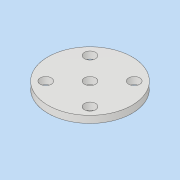
# Autodesk Inventor part: ServoHornDisc
Saved by Autodesk Inventor 2017.3 (Build 213256000, 256)
## iProperties
Created: 2016-11-02
Part Number: ServoHornDisc
Material: ABS Plastic
Document SubType Name: Modeling
Designer: techn
Density: 1.06 g/cm^3
Appearance: Smooth - White
Author: techn
Autodesk Inventor part; units mm, degrees
ref_plane "YZ Plane" through (0, 0, 0) normal (1, 0, 0) x (0, 1, 0)
ref_plane "XZ Plane" through (0, 0, 0) normal (0, 1, 0) x (-1, 0, 0)
ref_plane "XY Plane" through (0, 0, 0) normal (0, 0, 1) x (1, 0, 0)
sketch "Sketch1" plane through (0, 0, 0) normal (0, 1, 0) x (-1, 0, 0)
  circle A0 centre (0, 0) radius 2.8702
  dimension "d0" = 5.7404
  constraints: 1 centre point, 1 coincident
  measures "d0" diameter of A0
extrude "Extrusion1" add sketch "Sketch1" along normal blind 3.4036
sketch "Sketch6" plane through (0, 3.4036, 0) normal (0, 1, 0) x (1, 0, 0)
  circle A0 centre (0, 0) radius 11.938
  dimension "d22" = 23.876
  constraints: 1 centre point, 1 coincident
  measures "d22" diameter of A0
extrude "Extrusion8" add sketch "Sketch6" along normal mid plane 1.9939
sketch "Sketch7" plane through (0, 2.4067, 0) normal (0, -1, 0) x (1, 0, 0)
  circle A0 centre (0, 0) radius 4.445
  circle A1 centre (0, 0) radius 2.8702 projected
  circle A2 centre (0, 0) radius 1.5875
  dimension "d25" = 8.89
  dimension "d26" = 3.175
  constraints: 2 centre point, 2 coincident
  measures "d25" diameter of A0
  measures "d26" diameter of A2
extrude "Extrusion9" add sketch "Sketch7" along normal up to surface (2.4067 mm away) contours A0
extrude "Extrusion10" cut sketch "Sketch7" along normal through all contours A1 | A2
extrude "Extrusion11" cut sketch "Sketch7" against normal blind 1.9939 contours A2
sketch "Sketch8" plane through (0, 4.4006, 0) normal (0, 1, 0) x (1, 0, 0)
  line L0 (0, 0) -> (-6.2862, 6.2862)
  line L1 (0, 0) -> (8.89, 0) construction
  circle A0 centre (-6.2862, 6.2862) radius 1.5875
  circle A1 centre (-6.2862, -6.2862) radius 1.5875
  circle A2 centre (6.2862, -6.2862) radius 1.5875
  circle A3 centre (6.2862, 6.2862) radius 1.5875
  dimension "d33" = 8.89
  dimension "d34" = 135
  dimension "d35" = 3.175
  dimension "d38" = 360
  constraints: 4 centre point, 4 end point, 1 coincident, 1 equal length, 1 horizontal, 9 other
  measures "d33" distance of L0.start L0.end
  measures "d34" angle of L1 L0
  measures "d35" diameter of A0
extrude "Extrusion12" cut sketch "Sketch8" against normal blind 1.9939
body "Solid1"
